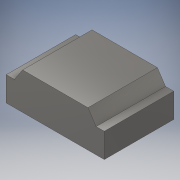
# Autodesk Inventor part: PiHDMI
Saved by Autodesk Inventor 2018 (Build 220112000, 112)
## iProperties
Created: 2018-01-13
Part Number: PiHDMI
Material: Stainless Steel
Document SubType Name: Modeling
Designer: Kyle-HP
Density: 8 g/cm^3
Appearance: Semi-Polished
Author: Kyle-HP
Autodesk Inventor part; units mm, degrees
ref_plane "YZ Plane" through (0, 0, 0) normal (1, 0, 0) x (0, 1, 0)
ref_plane "XZ Plane" through (0, 0, 0) normal (0, 1, 0) x (-1, 0, 0)
ref_plane "XY Plane" through (0, 0, 0) normal (0, 0, 1) x (1, 0, 0)
sketch "Sketch1" plane through (0, 0, 0) normal (0, 0, 1) x (1, 0, 0)
  line L0 (0, 0) -> (15.24, 0)
  line L1 (15.24, 0) -> (15.24, 3.81)
  line L2 (0, 0) -> (0, 3.81)
  line L3 (0, 3.81) -> (1.27, 3.81)
  line L4 (15.24, 3.81) -> (13.97, 3.81)
  line L5 (1.27, 3.81) -> (2.54, 5.715)
  line L6 (2.54, 5.715) -> (12.7, 5.715)
  line L7 (12.7, 5.715) -> (13.97, 3.81)
  dimension "d0" = 15.24
  dimension "d1" = 3.81
  dimension "d2" = 1.27
  dimension "d3" = 1.27
  dimension "d4" = 1.27
  dimension "d5" = 5.715
  dimension "d6" = 1.27
  constraints: 16 end point, 4 horizontal, 1 perpendicular, 1 vertical
  measures "d0" distance of L0.start L0.end
  measures "d1" distance of L0.end L1.end
  measures "d2" distance of L2.end L3.end
  measures "d3" distance of L1.end L4.end
  measures "d4" horizontal distance of L6.end L4.end
  measures "d5" distance from line of L0 L6.end
  measures "d6" horizontal distance of L3.end L5.end
extrude "Extrusion1" add sketch "Sketch1" along normal blind 10.795
body "Solid1"
